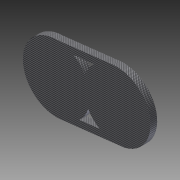
# Autodesk Inventor part: shooterchain2
Saved by Autodesk Inventor 2011 SP1 (Build 150282100, 282)
## iProperties
Created: 2012-01-20
Part Number: shooterchain2
Document SubType Name: Modeling
Designer: Christopher
Density: 1 g/cm^3
Author: Christopher
Autodesk Inventor part; units mm, degrees
ref_plane "YZ Plane" through (0, 0, 0) normal (1, 0, 0) x (0, 1, 0)
ref_plane "XZ Plane" through (0, 0, 0) normal (0, 1, 0) x (-1, 0, 0)
ref_plane "XY Plane" through (0, 0, 0) normal (0, 0, 1) x (1, 0, 0)
sketch "Sketch1" plane through (0, 0, 0) normal (0, 0, 1) x (1, 0, 0)
  circle A0 centre (68.7784, 0) radius 31.75
  circle A1 centre (125.9284, 6.35) radius 31.75
  line L0 (122.3086, 37.893) -> (68.7784, 31.75)
  line L1 (72.3981, -31.543) -> (133.1207, -24.5746)
  line L2 (85.1031, 27.2317) -> (104.1067, 29.4125)
  line L3 (109.6036, -20.8817) -> (90.6, -23.0625)
  line L4 (85.1031, 27.2317) -> (68.7784, 31.75)
  line L5 (90.6, -23.0625) -> (68.7784, -31.75)
  line L6 (109.6036, -20.8817) -> (125.9284, -25.4)
  line L7 (104.1067, 29.4125) -> (122.3086, 37.893)
  point P0 (0, 0)
  dimension "d0" = 57.15
  dimension "d1" = 6.35
  dimension "d2" = 63.5
  dimension "d3" = 63.5
  dimension "d4" = 6.35
  dimension "d5" = 6.35
  constraints: 16 end point, 11 point on circle, 3 parallel, 2 centre point, 2 coincident, 2 point on line, 1 tangent
  measures "d0" horizontal distance of point (125.928, 6.35) point (68.778, 0)
  measures "d1" vertical distance of point (68.778, 0) point (125.928, 6.35)
  measures "d2" diameter of A0
  measures "d3" diameter of A1
  measures "d4" distance between parallel lines of L1 L3
  measures "d5" distance between parallel lines of L0 L2
extrude "Extrusion1" add sketch "Sketch1" against normal blind 6.35 contours L4 A0 | A0 L0 A1 L2 | A0 A1 L5 L4 | A1 L7 L1 L6 A0 | A0 A1 | A1 L7 | L5 A0 | A0 L3 A1 L1 | L6 A1
body "Solid1"
